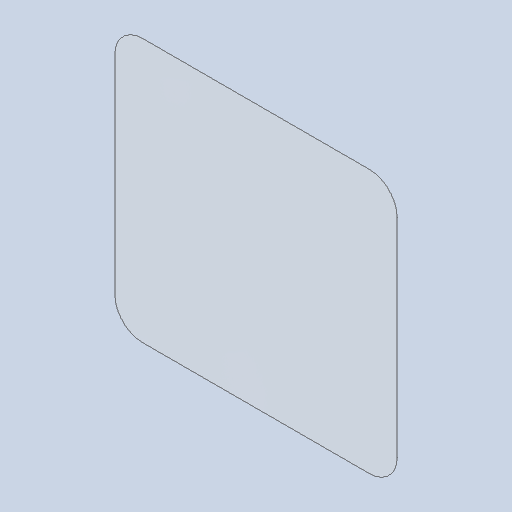
# Autodesk Inventor part: PLatico
Saved by Autodesk Inventor 2022.4 (Build 264492000, 492)
## iProperties
Created: 2022-11-28
Part Number: PLatico
Material: Plastic, Transparent
Document SubType Name: Modeling
Designer: David
Density: 1.188 g/cm^3
Appearance: Transparent - Clear
Author: David
Autodesk Inventor part; units mm, degrees
ref_plane "YZ Plane" through (0, 0, 0) normal (1, 0, 0) x (0, 1, 0)
ref_plane "XZ Plane" through (0, 0, 0) normal (0, 1, 0) x (-1, 0, 0)
ref_plane "XY Plane" through (0, 0, 0) normal (0, 0, 1) x (1, 0, 0)
sketch "Sketch1" plane through (0, 0, 0) normal (0, 0, 1) x (1, 0, 0)
  line L0 (-900, -850) -> (900, -850)
  line L1 (900, -850) -> (900, 850)
  line L2 (900, 850) -> (-900, 850)
  line L3 (-900, 850) -> (-900, -850)
  line L4 (-900, -850) -> (900, 850) construction
  line L5 (900, -850) -> (-900, 850) construction
  line L6 (-600, 700) -> (600, 700)
  line L7 (750, 550) -> (750, -550)
  line L8 (600, -700) -> (-600, -700)
  line L9 (-750, -550) -> (-750, 550)
  arc A0 (750, 550) -> (600, 700) centre (600, 550) ccw
  arc A1 (-600, 700) -> (-750, 550) centre (-600, 550) ccw
  arc A2 (-750, -550) -> (-600, -700) centre (-600, -550) ccw
  arc A3 (600, -700) -> (750, -550) centre (600, -550) ccw
  line L10 (600, 697) -> (-600, 697)
  arc A4 (-600, 697) -> (-747, 550) centre (-600, 550) ccw
  line L11 (-747, 550) -> (-747, -550)
  arc A5 (-747, -550) -> (-600, -697) centre (-600, -550) ccw
  line L12 (-600, -697) -> (600, -697)
  arc A6 (600, -697) -> (747, -550) centre (600, -550) ccw
  line L13 (747, -550) -> (747, 550)
  arc A7 (747, 550) -> (600, 697) centre (600, 550) ccw
  point P0 (0, 0)
  point P1 (0, 0)
  point P2 (0, 0)
  dimension "d0" = 1800
  dimension "d1" = 1700
  dimension "d2" = 150
  dimension "d3" = 150
  dimension "d4" = 150
  dimension "d5" = 150
  dimension "d6" = 150
  dimension "d7" = 3
  dimension "d10" = 1394
  constraints: 28 end point, 16 point on circle, 8 centre point, 8 tangent, 6 parallel, 3 perpendicular, 2 midpoint, 1 horizontal, 10 other
  measures "d0" distance of L2.end L1.end
  measures "d1" distance of L1.end L0.end
  measures "d2" distance between parallel lines of L2 L6
  measures "d3" radius of A0
  measures "d4" radius of A1
  measures "d5" radius of A2
  measures "d6" radius of A3
  measures "d7" distance between parallel lines of L6 L10
  measures "d10" distance between parallel lines of L12 L10
extrude "Extrusion1" add sketch "Sketch1" along normal mid plane 2 contours A7 L13 A6 L12 A5 L11 A4 L10
equation "\"Space6\" = 0"
equation "\"Space7\" = 0"
body "Solid1"
